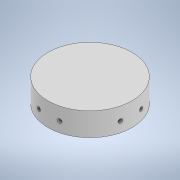
# Autodesk Inventor part: acople pinza
Saved by Autodesk Inventor 2021 (Build 250183000, 183)
## iProperties
Created: 2022-04-17
Part Number: acople pinza
Material: Genérico
Document SubType Name: Modeling
Designer: orgyn
Density: 1 g/cm^3
Appearance: Valor por defecto
Author: orgyn
Autodesk Inventor part; units mm, degrees
ref_plane "YZ Plane" through (0, 0, 0) normal (1, 0, 0) x (0, 1, 0)
ref_plane "XZ Plane" through (0, 0, 0) normal (0, 1, 0) x (-1, 0, 0)
ref_plane "XY Plane" through (0, 0, 0) normal (0, 0, 1) x (1, 0, 0)
sketch "Boceto1" plane through (0, 0, 0) normal (0, 1, 0) x (-1, 0, 0)
  circle A0 centre (0, 0) radius 32.5
  line L0 (0, 0) -> (22.5, 0)
  line L1 (22.5, 0) -> (22.5, -16)
  line L2 (22.5, -16) -> (22.5, 16)
  line L3 (0, 0) -> (0, 22.5)
  line L4 (0, 22.5) -> (16, 22.5)
  line L5 (16, 22.5) -> (-16, 22.5)
  line L6 (0, 0) -> (-22.5, 0)
  line L7 (-22.5, 0) -> (-22.5, 16)
  line L8 (-22.5, 16) -> (-22.5, -16)
  line L9 (0, 0) -> (0, -22.5)
  line L10 (0, -22.5) -> (-16, -22.5)
  line L11 (-16, -22.5) -> (16, -22.5)
  line L12 (22.5, 16) -> (16, 22.5)
  line L13 (-16, 22.5) -> (-22.5, 16)
  line L14 (-22.5, -16) -> (-16, -22.5)
  line L15 (16, -22.5) -> (22.5, -16)
  dimension "d0" = 65
  dimension "d1" = 22.5
  dimension "d3" = 16
  dimension "d4" = 32
  dimension "d7" = 360
  constraints: 32 end point, 5 point on line, 3 perpendicular, 1 centre point, 1 coincident, 1 horizontal, 1 vertical, 29 other
  measures "d0" diameter of A0
  measures "d1" distance of L0.start L0.end
  measures "d3" distance of L0.end L1.end
  measures "d4" distance of L1.end L2.end
extrude "Extrusión1" add sketch "Boceto1" along normal blind 15
sketch "Boceto2" plane through (-16, 0, -22.5) normal (0, 0, 1) x (1, 0, 0)
  line L0 (16, 0) -> (16, 8)
  line L1 (16, 8) -> (24, 8)
  line L2 (24, 8) -> (8, 8)
  circle A0 centre (8, 8) radius 1.5
  circle A1 centre (24, 8) radius 1.5
  dimension "d11" = 8
  dimension "d12" = 8
  dimension "d13" = 16
  dimension "d15" = 3
  dimension "d16" = 3
  constraints: 6 end point, 2 centre point, 2 coincident, 1 horizontal, 1 point on line, 1 vertical
  measures "d11" distance of L0.start L0.end
  measures "d12" distance of L0.end L1.end
  measures "d13" distance of L1.end L2.end
  measures "d15" diameter of A0
  measures "d16" diameter of A1
extrude "Extrusión2" cut sketch "Boceto2" along normal mid plane 10200
sketch "Boceto3" plane through (22.5, 0, -16) normal (-1, 0, 0) x (0, 0, 1)
  line L0 (16, 0) -> (16, 8)
  line L1 (16, 8) -> (24, 8)
  line L2 (24, 8) -> (8, 8)
  circle A0 centre (8, 8) radius 1.5
  circle A1 centre (24, 8) radius 1.5
  dimension "d19" = 8
  dimension "d20" = 8
  dimension "d21" = 16
  dimension "d22" = 3
  dimension "d23" = 3
  constraints: 6 end point, 2 centre point, 2 coincident, 1 perpendicular, 1 point on line, 1 vertical
  measures "d19" distance of L0.start L0.end
  measures "d20" distance of L0.end L1.end
  measures "d21" distance of L1.end L2.end
  measures "d22" diameter of A0
  measures "d23" diameter of A1
extrude "Extrusión3" cut sketch "Boceto3" against normal mid plane 10200
sketch "Boceto4" plane through (0, 15, 0) normal (0, 1, 0) x (1, 0, 0)
  circle A0 centre (0, 0) radius 32.5
  constraints: 1 centre point, 1 coincident
extrude "Extrusión4" add sketch "Boceto4" along normal blind 3
